Autodesk Fusion 360 part; units mm, degrees
(part 2 of 2)
sketch "スケッチ20" plane through (0, 0, 39.9) normal (0, 0, 1) x (1, 0, 0) in component "CASE_LID_print"
  line L0 (0.01, -5.9596) -> (0.01, -3.5388)
  line L1 (0.01, -3.5388) -> (1.0436, -3.5388)
  line L2 (1.0436, -3.5388) -> (1.0436, -3.8652)
  line L3 (1.0436, -3.8652) -> (0.3568, -3.8652)
  line L4 (0.3568, -3.8652) -> (0.3568, -4.5758)
  line L5 (0.3568, -4.5758) -> (0.9552, -4.5758)
  line L6 (0.9552, -4.5758) -> (0.9552, -4.9022)
  line L7 (0.9552, -4.9022) -> (0.3568, -4.9022)
  line L8 (0.3568, -4.9022) -> (0.3568, -5.6128)
  line L9 (0.3568, -5.6128) -> (1.0436, -5.6128)
  line L10 (1.0436, -5.6128) -> (1.0436, -5.9596)
  line L11 (1.0436, -5.9596) -> (0.01, -5.9596)
  line L12 (1.268, -5.9596) -> (1.268, -3.5388)
  line L13 (1.268, -3.5388) -> (1.6012, -3.5388)
  line L14 (1.6012, -3.5388) -> (2.0466, -4.8206)
  line L15 (2.0466, -4.8206) -> (2.0534, -4.8206)
  line L16 (2.0534, -4.8206) -> (2.4954, -3.5388)
  line L17 (2.4954, -3.5388) -> (2.832, -3.5388)
  line L18 (2.832, -3.5388) -> (2.832, -5.9596)
  line L19 (2.832, -5.9596) -> (2.4852, -5.9596)
  line L20 (2.4852, -5.9596) -> (2.4852, -4.4874)
  line L21 (2.4852, -4.4874) -> (2.4784, -4.4874)
  line L22 (2.4784, -4.4874) -> (2.135, -5.5278)
  line L23 (2.135, -5.5278) -> (1.9616, -5.5278)
  line L24 (1.9616, -5.5278) -> (1.6216, -4.4874)
  line L25 (1.6216, -4.4874) -> (1.6148, -4.4874)
  line L26 (1.6148, -4.4874) -> (1.6148, -5.9596)
  line L27 (1.6148, -5.9596) -> (1.268, -5.9596)
  line L28 (3.1584, -5.9596) -> (3.1584, -3.5388)
  line L29 (3.1584, -3.5388) -> (4.192, -3.5388)
  line L30 (4.192, -3.5388) -> (4.192, -3.8652)
  line L31 (4.192, -3.8652) -> (3.5052, -3.8652)
  line L32 (3.5052, -3.8652) -> (3.5052, -4.5758)
  line L33 (3.5052, -4.5758) -> (4.1036, -4.5758)
  line L34 (4.1036, -4.5758) -> (4.1036, -4.9022)
  line L35 (4.1036, -4.9022) -> (3.5052, -4.9022)
  line L36 (3.5052, -4.9022) -> (3.5052, -5.6128)
  line L37 (3.5052, -5.6128) -> (4.192, -5.6128)
  line L38 (4.192, -5.6128) -> (4.192, -5.9596)
  line L39 (4.192, -5.9596) -> (3.1584, -5.9596)
  line L40 (4.7632, -3.8652) -> (4.7632, -4.62)
  line L41 (4.7632, -4.62) -> (4.9604, -4.62)
  spline S0 degree 3 poles (4.9604, -4.62) (4.9881, -4.6195) (5.0381, -4.6187) (5.0855, -4.6031) (5.1066, -4.5962) knots 0 0 0 0 0.008266 0.014887 0.014887 0.014887 0.014887
  spline S1 degree 3 poles (5.1066, -4.5962) (5.1236, -4.5864) (5.1571, -4.5673) (5.1802, -4.5365) (5.1916, -4.5214) knots 0 0 0 0 0.005823 0.011428 0.011428 0.011428 0.011428
  spline S2 degree 3 poles (5.1916, -4.5214) (5.2, -4.5041) (5.218, -4.4674) (5.2252, -4.4271) (5.229, -4.4058) knots 0 0 0 0 0.005748 0.012202 0.012202 0.012202 0.012202
  spline S3 degree 3 poles (5.229, -4.4058) (5.232, -4.3803) (5.2383, -4.3261) (5.2389, -4.2715) (5.2392, -4.2426) knots 0 0 0 0 0.007688 0.016362 0.016362 0.016362 0.016362
  spline S4 degree 3 poles (5.2392, -4.2426) (5.2389, -4.2139) (5.2384, -4.1605) (5.232, -4.1074) (5.229, -4.0828) knots 0 0 0 0 0.008589 0.016023 0.016023 0.016023 0.016023
  spline S5 degree 3 poles (5.229, -4.0828) (5.225, -4.0603) (5.2174, -4.0175) (5.1976, -3.9788) (5.1882, -3.9604) knots 0 0 0 0 0.006804 0.012967 0.012967 0.012967 0.012967
  spline S6 degree 3 poles (5.1882, -3.9604) (5.1587, -3.9328) (5.0907, -3.8691) (4.9966, -3.8666) (4.9434, -3.8652) knots 0 0 0 0 0.011764 0.02708 0.02708 0.02708 0.02708
  line L42 (4.9434, -3.8652) -> (4.7632, -3.8652)
  line L43 (4.4164, -5.9596) -> (4.4164, -3.5388)
  line L44 (4.4164, -3.5388) -> (4.974, -3.5388)
  spline S7 degree 3 poles (4.974, -3.5388) (5.1523, -3.5749) (5.5316, -3.6516) (5.5671, -4.0424) (5.586, -4.2494) knots 0 0 0 0 0.049218 0.104666 0.104666 0.104666 0.104666
  spline S8 degree 3 poles (5.586, -4.2494) (5.584, -4.3161) (5.5803, -4.4411) (5.5378, -4.5585) (5.518, -4.6132) knots 0 0 0 0 0.019878 0.03722 0.03722 0.03722 0.03722
  spline S9 degree 3 poles (5.518, -4.6132) (5.4911, -4.6612) (5.435, -4.7615) (5.3376, -4.8227) (5.2868, -4.8546) knots 0 0 0 0 0.016243 0.033906 0.033906 0.033906 0.033906
  line L45 (5.2868, -4.8546) -> (5.6608, -5.9596)
  line L46 (5.6608, -5.9596) -> (5.2936, -5.9596)
  line L47 (5.2936, -5.9596) -> (4.9706, -4.926)
  line L48 (4.9706, -4.926) -> (4.7632, -4.926)
  line L49 (4.7632, -4.926) -> (4.7632, -5.9596)
  line L50 (4.7632, -5.9596) -> (4.4164, -5.9596)
  spline S10 degree 3 poles (5.8444, -4.11) (5.8461, -4.0636) (5.8494, -3.9747) (5.8805, -3.8914) (5.8954, -3.8516) knots 0 0 0 0 0.013829 0.02649 0.02649 0.02649 0.02649
  spline S11 degree 3 poles (5.8954, -3.8516) (5.9135, -3.816) (5.9489, -3.7465) (6.0043, -3.6915) (6.0314, -3.6646) knots 0 0 0 0 0.011882 0.023255 0.023255 0.023255 0.023255
  spline S12 degree 3 poles (6.0314, -3.6646) (6.0595, -3.6422) (6.1156, -3.5974) (6.1819, -3.5697) (6.215, -3.5558) knots 0 0 0 0 0.010711 0.021434 0.021434 0.021434 0.021434
  spline S13 degree 3 poles (6.215, -3.5558) (6.2499, -3.5449) (6.3185, -3.5234) (6.3904, -3.5201) (6.4258, -3.5184) knots 0 0 0 0 0.010907 0.021488 0.021488 0.021488 0.021488
  spline S14 degree 3 poles (6.4258, -3.5184) (6.4609, -3.52) (6.5317, -3.5232) (6.5992, -3.5449) (6.6332, -3.5558) knots 0 0 0 0 0.010497 0.021157 0.021157 0.021157 0.021157
  spline S15 degree 3 poles (6.6332, -3.5558) (6.6675, -3.5697) (6.7358, -3.5973) (6.7944, -3.6422) (6.8236, -3.6646) knots 0 0 0 0 0.01103 0.022019 0.022019 0.022019 0.022019
  spline S16 degree 3 poles (6.8236, -3.6646) (6.8497, -3.6916) (6.9035, -3.7471) (6.9383, -3.8161) (6.9562, -3.8516) knots 0 0 0 0 0.011203 0.023042 0.023042 0.023042 0.023042
  spline S17 degree 3 poles (6.9562, -3.8516) (6.9711, -3.8914) (7.0022, -3.9747) (7.0055, -4.0636) (7.0072, -4.11) knots 0 0 0 0 0.012662 0.02649 0.02649 0.02649 0.02649
  line L51 (7.0072, -4.11) -> (7.0072, -4.2324)
  line L52 (7.0072, -4.2324) -> (6.6604, -4.2324)
  line L53 (6.6604, -4.2324) -> (6.6604, -4.11)
  spline S18 degree 3 poles (6.6604, -4.11) (6.6587, -4.072) (6.6555, -4.0023) (6.6098, -3.9501) (6.589, -3.9264) knots 0 0 0 0 0.011025 0.020225 0.020225 0.020225 0.020225
  spline S19 degree 3 poles (6.589, -3.9264) (6.565, -3.9086) (6.5166, -3.8725) (6.4563, -3.8676) (6.4258, -3.8652) knots 0 0 0 0 0.008776 0.017747 0.017747 0.017747 0.017747
  spline S20 degree 3 poles (6.4258, -3.8652) (6.3951, -3.8677) (6.3339, -3.8727) (6.284, -3.9086) (6.2592, -3.9264) knots 0 0 0 0 0.009055 0.01805 0.01805 0.01805 0.01805
  spline S21 degree 3 poles (6.2592, -3.9264) (6.2394, -3.9502) (6.1956, -4.0031) (6.1927, -4.0721) (6.1912, -4.11) knots 0 0 0 0 0.009053 0.020065 0.020065 0.020065 0.020065
  line L54 (6.1912, -4.11) -> (6.1912, -5.3884)
  spline S22 degree 3 poles (6.1912, -5.3884) (6.1929, -5.4265) (6.1959, -5.4964) (6.2394, -5.5507) (6.2592, -5.5754) knots 0 0 0 0 0.011096 0.020361 0.020361 0.020361 0.020361
  spline S23 degree 3 poles (6.2592, -5.5754) (6.2841, -5.5923) (6.3345, -5.6263) (6.3952, -5.6309) (6.4258, -5.6332) knots 0 0 0 0 0.008867 0.017908 0.017908 0.017908 0.017908
  spline S24 degree 3 poles (6.4258, -5.6332) (6.4562, -5.631) (6.5159, -5.6266) (6.5649, -5.5923) (6.589, -5.5754) knots 0 0 0 0 0.008957 0.017603 0.017603 0.017603 0.017603
  spline S25 degree 3 poles (6.589, -5.5754) (6.6098, -5.5508) (6.6551, -5.4972) (6.6585, -5.4266) (6.6604, -5.3884) knots 0 0 0 0 0.009408 0.020517 0.020517 0.020517 0.020517
  line L55 (6.6604, -5.3884) -> (6.6604, -4.9328)
  line L56 (6.6604, -4.9328) -> (6.385, -4.9328)
  line L57 (6.385, -4.9328) -> (6.385, -4.6268)
  line L58 (6.385, -4.6268) -> (7.0072, -4.6268)
  line L59 (7.0072, -4.6268) -> (7.0072, -5.3884)
  spline S26 degree 3 poles (7.0072, -5.3884) (7.0057, -5.4363) (7.0028, -5.5264) (6.9711, -5.6107) (6.9562, -5.6502) knots 0 0 0 0 0.014252 0.026833 0.026833 0.026833 0.026833
  spline S27 degree 3 poles (6.9562, -5.6502) (6.9383, -5.6846) (6.9034, -5.7515) (6.8497, -5.8046) (6.8236, -5.8304) knots 0 0 0 0 0.011546 0.022495 0.022495 0.022495 0.022495
  spline S28 degree 3 poles (6.8236, -5.8304) (6.7945, -5.8538) (6.7364, -5.9003) (6.6675, -5.9285) (6.6332, -5.9426) knots 0 0 0 0 0.011136 0.022202 0.022202 0.022202 0.022202
  spline S29 degree 3 poles (6.6332, -5.9426) (6.5992, -5.9535) (6.5317, -5.9752) (6.4609, -5.9784) (6.4258, -5.98) knots 0 0 0 0 0.010661 0.021157 0.021157 0.021157 0.021157
  spline S30 degree 3 poles (6.4258, -5.98) (6.3904, -5.9783) (6.3185, -5.975) (6.2499, -5.9535) (6.215, -5.9426) knots 0 0 0 0 0.010581 0.021488 0.021488 0.021488 0.021488
  spline S31 degree 3 poles (6.215, -5.9426) (6.1818, -5.9285) (6.115, -5.9002) (6.0594, -5.8537) (6.0314, -5.8304) knots 0 0 0 0 0.010759 0.021622 0.021622 0.021622 0.021622
  spline S32 degree 3 poles (6.0314, -5.8304) (6.0043, -5.8047) (5.949, -5.7522) (5.9135, -5.6847) (5.8954, -5.6502) knots 0 0 0 0 0.011123 0.022712 0.022712 0.022712 0.022712
  spline S33 degree 3 poles (5.8954, -5.6502) (5.8805, -5.6107) (5.8488, -5.5264) (5.8459, -5.4363) (5.8444, -5.3884) knots 0 0 0 0 0.012581 0.026833 0.026833 0.026833 0.026833
  line L60 (5.8444, -5.3884) -> (5.8444, -4.11)
  line L61 (7.3132, -5.9596) -> (7.3132, -3.5388)
  line L62 (7.3132, -3.5388) -> (8.3468, -3.5388)
  line L63 (8.3468, -3.5388) -> (8.3468, -3.8652)
  line L64 (8.3468, -3.8652) -> (7.66, -3.8652)
  line L65 (7.66, -3.8652) -> (7.66, -4.5758)
  line L66 (7.66, -4.5758) -> (8.2584, -4.5758)
  line L67 (8.2584, -4.5758) -> (8.2584, -4.9022)
  line L68 (8.2584, -4.9022) -> (7.66, -4.9022)
  line L69 (7.66, -4.9022) -> (7.66, -5.6128)
  line L70 (7.66, -5.6128) -> (8.3468, -5.6128)
  line L71 (8.3468, -5.6128) -> (8.3468, -5.9596)
  line L72 (8.3468, -5.9596) -> (7.3132, -5.9596)
  line L73 (8.5576, -5.9596) -> (8.5576, -3.5388)
  line L74 (8.5576, -3.5388) -> (8.8908, -3.5388)
  line L75 (8.8908, -3.5388) -> (9.4144, -4.9974)
  line L76 (9.4144, -4.9974) -> (9.4212, -4.9974)
  line L77 (9.4212, -4.9974) -> (9.4212, -3.5388)
  line L78 (9.4212, -3.5388) -> (9.768, -3.5388)
  line L79 (9.768, -3.5388) -> (9.768, -5.9596)
  line L80 (9.768, -5.9596) -> (9.4416, -5.9596)
  line L81 (9.4416, -5.9596) -> (8.9112, -4.5044)
  line L82 (8.9112, -4.5044) -> (8.9044, -4.5044)
  line L83 (8.9044, -4.5044) -> (8.9044, -5.9596)
  line L84 (8.9044, -5.9596) -> (8.5576, -5.9596)
  line L85 (11.1824, -5.2694) -> (11.1824, -5.419)
  spline S34 degree 3 poles (11.1824, -5.419) (11.1806, -5.4559) (11.1769, -5.5296) (11.1511, -5.5987) (11.1382, -5.6332) knots 0 0 0 0 0.011021 0.021988 0.021988 0.021988 0.021988
  spline S35 degree 3 poles (11.1382, -5.6332) (11.1231, -5.6653) (11.0929, -5.7296) (11.0461, -5.7831) (11.0226, -5.81) knots 0 0 0 0 0.01057 0.021217 0.021217 0.021217 0.021217
  spline S36 degree 3 poles (11.0226, -5.81) (10.9964, -5.8349) (10.9434, -5.8851) (10.8785, -5.9188) (10.8458, -5.9358) knots 0 0 0 0 0.010787 0.021794 0.021794 0.021794 0.021794
  spline S37 degree 3 poles (10.8458, -5.9358) (10.8119, -5.9487) (10.7429, -5.9749) (10.6691, -5.9783) (10.6316, -5.98) knots 0 0 0 0 0.010806 0.021996 0.021996 0.021996 0.021996
  spline S38 degree 3 poles (10.6316, -5.98) (10.5983, -5.9788) (10.5306, -5.9763) (10.4646, -5.9607) (10.431, -5.9528) knots 0 0 0 0 0.009968 0.020287 0.020287 0.020287 0.020287
  spline S39 degree 3 poles (10.431, -5.9528) (10.3978, -5.942) (10.3314, -5.9204) (10.2754, -5.8786) (10.2474, -5.8576) knots 0 0 0 0 0.010387 0.020807 0.020807 0.020807 0.020807
  spline S40 degree 3 poles (10.2474, -5.8576) (10.2211, -5.8329) (10.1669, -5.7821) (10.1303, -5.7174) (10.1114, -5.6842) knots 0 0 0 0 0.01076 0.022149 0.022149 0.022149 0.022149
  spline S41 degree 3 poles (10.1114, -5.6842) (10.0966, -5.6435) (10.0641, -5.5547) (10.0617, -5.4601) (10.0604, -5.4088) knots 0 0 0 0 0.012905 0.028173 0.028173 0.028173 0.028173
  line L86 (10.0604, -5.4088) -> (10.0604, -4.076)
  spline S42 degree 3 poles (10.0604, -4.076) (10.062, -4.0374) (10.065, -3.9618) (10.0893, -3.8901) (10.1012, -3.855) knots 0 0 0 0 0.01152 0.022577 0.022577 0.022577 0.022577
  spline S43 degree 3 poles (10.1012, -3.855) (10.1161, -3.8223) (10.1456, -3.7574) (10.1932, -3.7044) (10.2168, -3.6782) knots 0 0 0 0 0.010721 0.021235 0.021235 0.021235 0.021235
  spline S44 degree 3 poles (10.2168, -3.6782) (10.243, -3.6546) (10.296, -3.607) (10.3609, -3.5775) (10.3936, -3.5626) knots 0 0 0 0 0.010514 0.021235 0.021235 0.021235 0.021235
  spline S45 degree 3 poles (10.3936, -3.5626) (10.4301, -3.5497) (10.5049, -3.5233) (10.5842, -3.5201) (10.6248, -3.5184) knots 0 0 0 0 0.011537 0.023657 0.023657 0.023657 0.023657
  spline S46 degree 3 poles (10.6248, -3.5184) (10.7018, -3.5243) (10.8515, -3.5357) (10.9667, -3.6316) (11.0226, -3.6782) knots 0 0 0 0 0.022542 0.043831 0.043831 0.043831 0.043831
  spline S47 degree 3 poles (11.0226, -3.6782) (11.0462, -3.7059) (11.0944, -3.7622) (11.1234, -3.8305) (11.1382, -3.8652) knots 0 0 0 0 0.010847 0.0221 0.0221 0.0221 0.0221
  spline S48 degree 3 poles (11.1382, -3.8652) (11.1511, -3.9017) (11.1775, -3.9765) (11.1807, -4.0558) (11.1824, -4.0964) knots 0 0 0 0 0.011536 0.023657 0.023657 0.023657 0.023657
  line L87 (11.1824, -4.0964) -> (11.1824, -4.2324)
  line L88 (11.1824, -4.2324) -> (10.8356, -4.2324)
  line L89 (10.8356, -4.2324) -> (10.8356, -4.1168)
  spline S49 degree 3 poles (10.8356, -4.1168) (10.8334, -4.0842) (10.8291, -4.0203) (10.7947, -3.9664) (10.7778, -3.94) knots 0 0 0 0 0.009629 0.018869 0.018869 0.018869 0.018869
  spline S50 degree 3 poles (10.7778, -3.94) (10.7566, -3.9182) (10.7138, -3.874) (10.6524, -3.8682) (10.6214, -3.8652) knots 0 0 0 0 0.008815 0.017851 0.017851 0.017851 0.017851
  spline S51 degree 3 poles (10.6214, -3.8652) (10.5829, -3.867) (10.5129, -3.8702) (10.4681, -3.9231) (10.448, -3.9468) knots 0 0 0 0 0.010986 0.019947 0.019947 0.019947 0.019947
  spline S52 degree 3 poles (10.448, -3.9468) (10.4361, -3.9762) (10.4102, -4.0404) (10.4082, -4.1098) (10.4072, -4.1474) knots 0 0 0 0 0.009435 0.020617 0.020617 0.020617 0.020617
  line L90 (10.4072, -4.1474) -> (10.4072, -5.385)
  spline S53 degree 3 poles (10.4072, -5.385) (10.4086, -5.4179) (10.4111, -5.48) (10.4385, -5.5356) (10.4514, -5.5618) knots 0 0 0 0 0.009753 0.018403 0.018403 0.018403 0.018403
  spline S54 degree 3 poles (10.4514, -5.5618) (10.4719, -5.5826) (10.5172, -5.6286) (10.5823, -5.6316) (10.618, -5.6332) knots 0 0 0 0 0.008456 0.018728 0.018728 0.018728 0.018728
  spline S55 degree 3 poles (10.618, -5.6332) (10.6297, -5.6327) (10.6538, -5.6317) (10.6773, -5.626) (10.6894, -5.623) knots 0 0 0 0 0.003494 0.007229 0.007229 0.007229 0.007229
  spline S56 degree 3 poles (10.6894, -5.623) (10.7027, -5.6179) (10.7295, -5.6076) (10.7526, -5.5907) (10.7642, -5.5822) knots 0 0 0 0 0.004264 0.008554 0.008554 0.008554 0.008554
  spline S57 degree 3 poles (10.7642, -5.5822) (10.7742, -5.5719) (10.7953, -5.5498) (10.8083, -5.5221) (10.8152, -5.5074) knots 0 0 0 0 0.004278 0.009108 0.009108 0.009108 0.009108
  spline S58 degree 3 poles (10.8152, -5.5074) (10.8211, -5.4897) (10.8341, -5.4511) (10.8351, -5.4104) (10.8356, -5.3884) knots 0 0 0 0 0.005569 0.012134 0.012134 0.012134 0.012134
  line L91 (10.8356, -5.3884) -> (10.8356, -5.2694)
  line L92 (10.8356, -5.2694) -> (11.1824, -5.2694)
  line L93 (11.7876, -5.9596) -> (11.7876, -4.9362)
  line L94 (11.7876, -4.9362) -> (11.3116, -3.5388)
  line L95 (11.3116, -3.5388) -> (11.6788, -3.5388)
  line L96 (11.6788, -3.5388) -> (11.9576, -4.501)
  line L97 (11.9576, -4.501) -> (11.9644, -4.501)
  line L98 (11.9644, -4.501) -> (12.2432, -3.5388)
  line L99 (12.2432, -3.5388) -> (12.6104, -3.5388)
  line L100 (12.6104, -3.5388) -> (12.1344, -4.9362)
  line L101 (12.1344, -4.9362) -> (12.1344, -5.9596)
  line L102 (12.1344, -5.9596) -> (11.7876, -5.9596)
extrude "押し出し39" add sketch "スケッチ20" along normal blind 0.8 separate body contours L0 L1 L2 L3 L4 L5 L6 L7 L8 L9 L10 L11 makes body 57 in component "CASE_LID_print"
extrude "押し出し40" add sketch "スケッチ20" along normal blind 0.8 separate body contours S10 S11 S12 S13 S14 S15 S16 S17 L51 L52 L53 S18 S19 S20 S21 L54 S22 S23 S24 S25 L55 L56 L57 L58 L59 S26 S27 S28 S29 S30 S31 S32 S33 L60 makes body 58 in component "CASE_LID_print"
extrude "押し出し41" add sketch "スケッチ20" along normal blind 0.8 separate body contours L61 L62 L63 L64 L65 L66 L67 L68 L69 L70 L71 L72 makes body 59 in component "CASE_LID_print"
extrude "押し出し42" add sketch "スケッチ20" along normal blind 0.8 separate body contours L40 L41 S0 S1 S2 S3 S4 S5 S6 L42 makes body 60 in component "CASE_LID_print"
extrude "押し出し43" add sketch "スケッチ20" along normal blind 0.8 separate body contours L43 L44 S7 S8 S9 L45 L46 L47 L48 L49 L50 makes body 61 in component "CASE_LID_print"
extrude "押し出し44" add sketch "スケッチ20" along normal blind 0.8 separate body contours L73 L74 L75 L76 L77 L78 L79 L80 L81 L82 L83 L84 makes body 62 in component "CASE_LID_print"
extrude "押し出し45" add sketch "スケッチ20" along normal blind 0.8 separate body contours L28 L29 L30 L31 L32 L33 L34 L35 L36 L37 L38 L39 makes body 63 in component "CASE_LID_print"
extrude "押し出し46" add sketch "スケッチ20" along normal blind 0.8 separate body contours L85 S34 S35 S36 S37 S38 S39 S40 S41 L86 S42 S43 S44 S45 S46 S47 S48 L87 L88 L89 S49 S50 S51 S52 L90 S53 S54 S55 S56 S57 S58 L91 L92 makes body 64 in component "CASE_LID_print"
extrude "押し出し47" add sketch "スケッチ20" along normal blind 0.8 separate body contours L12 L13 L14 L15 L16 L17 L18 L19 L20 L21 L22 L23 L24 L25 L26 L27 makes body 65 in component "CASE_LID_print"
extrude "押し出し48" add sketch "スケッチ20" along normal blind 0.8 separate body contours L93 L94 L95 L96 L97 L98 L99 L100 L101 L102 makes body 66 in component "CASE_LID_print"
move_body "移動2'" bodies 57 58 59 60 61 62 63 64 65 66 to x (1, 0, 0) y (0, 1, 0) z (0, 0, 1) at (-0.3102, 5.0492, 0) in component "CASE_LID_print"
combine "結合12'" operation add target body 19 tool bodies 57 58 59 60 61 62 63 64 65 66 in component "CASE_LID_print"
ref_plane "作業平面21" through (0, 0, 32.5) normal (0, 0, 1) x (1, 0, 0) in component "CASE_LID_print"
sketch "スケッチ21" plane through (0, 0, 32.5) normal (0, 0, 1) x (1, 0, 0) in component "CASE_LID_print"
  circle A0 centre (6, -18) radius 5.25
extrude "押し出し49" add sketch "スケッチ21" along normal blind 8.45 separate body makes body 67 in component "CASE_LID_print"
ref_plane "作業平面22" through (0, 0, 35) normal (0, 0, 1) x (1, 0, 0) in component "CASE_LID_print"
sketch "スケッチ22" plane through (0, 0, 35) normal (0, 0, 1) x (1, 0, 0) in component "CASE_LID_print"
  circle A0 centre (6, -18) radius 9.9
extrude "押し出し50" add sketch "スケッチ22" along normal blind 5.95 separate body makes body 68 in component "CASE_LID_print"
combine "結合13" operation cut target body 19 tool bodies 67 68 in component "CASE_LID_print"
ref_plane "作業平面1" through (0, 0, 37.6) normal (0, 0, 1) x (1, 0, 0) in component "EMERGENCY_BUTTON_PLUNGER_print"
sketch "スケッチ1 (3)" plane through (0, 0, 37.6) normal (0, 0, 1) x (1, 0, 0) in component "EMERGENCY_BUTTON_PLUNGER_print"
  circle A0 centre (6, -18) radius 9
extrude "押し出し1''" add sketch "スケッチ1 (3)" along normal blind 4 separate body makes body 69 in component "EMERGENCY_BUTTON_PLUNGER_print"
ref_plane "作業平面2" through (0, 0, 21.65) normal (0, 0, 1) x (1, 0, 0) in component "EMERGENCY_BUTTON_PLUNGER_print"
sketch "スケッチ2 (3)" plane through (0, 0, 21.65) normal (0, 0, 1) x (1, 0, 0) in component "EMERGENCY_BUTTON_PLUNGER_print"
  circle A0 centre (6, -18) radius 3.5
extrude "押し出し2''" add sketch "スケッチ2 (3)" along normal blind 15.95 separate body makes body 70 in component "EMERGENCY_BUTTON_PLUNGER_print"
combine "結合1''" operation add target body 69 tool bodies 70 in component "EMERGENCY_BUTTON_PLUNGER_print"
ref_plane "作業平面3" through (0, 0, 41.55) normal (0, 0, 1) x (1, 0, 0) in component "EMERGENCY_BUTTON_PLUNGER_print"
sketch "スケッチ3 (3)" plane through (0, 0, 41.55) normal (0, 0, 1) x (1, 0, 0) in component "EMERGENCY_BUTTON_PLUNGER_print"
  circle A0 centre (6, -18) radius 6.7
extrude "押し出し3''" add sketch "スケッチ3 (3)" along normal blind 0.55 separate body makes body 71 in component "EMERGENCY_BUTTON_PLUNGER_print"
ref_plane "作業平面4" through (0, 0, 41.45) normal (0, 0, 1) x (1, 0, 0) in component "EMERGENCY_BUTTON_PLUNGER_print"
sketch "スケッチ4 (3)" plane through (0, 0, 41.45) normal (0, 0, 1) x (1, 0, 0) in component "EMERGENCY_BUTTON_PLUNGER_print"
  circle A0 centre (6, -18) radius 5.2
extrude "押し出し4''" add sketch "スケッチ4 (3)" along normal blind 0.85 separate body makes body 72 in component "EMERGENCY_BUTTON_PLUNGER_print"
combine "結合2''" operation cut target body 71 tool bodies 72 in component "EMERGENCY_BUTTON_PLUNGER_print"
combine "結合3''" operation add target body 69 tool bodies 71 in component "EMERGENCY_BUTTON_PLUNGER_print"
ref_plane "作業平面5" through (0, 0, 41.55) normal (0, 0, 1) x (1, 0, 0) in component "EMERGENCY_BUTTON_PLUNGER_print"
sketch "スケッチ5 (3)" plane through (0, 0, 41.55) normal (0, 0, 1) x (1, 0, 0) in component "EMERGENCY_BUTTON_PLUNGER_print"
  line L0 (1.3541, -16.4787) -> (1.1543, -20.1691)
  line L1 (1.1543, -20.1691) -> (0.2098, -20.1691)
  line L2 (0.2098, -20.1691) -> (0.01, -16.4787)
  line L3 (0.01, -16.4787) -> (1.3541, -16.4787)
  line L4 (1.2542, -20.3991) -> (1.2542, -21.38)
  line L5 (1.2542, -21.38) -> (0.1099, -21.38)
  line L6 (0.1099, -21.38) -> (0.1099, -20.3991)
  line L7 (0.1099, -20.3991) -> (1.2542, -20.3991)
extrude "押し出し5''" add sketch "スケッチ5 (3)" along normal blind 0.6 separate body contours L0 L1 L2 L3 makes body 73 in component "EMERGENCY_BUTTON_PLUNGER_print"
extrude "押し出し6''" add sketch "スケッチ5 (3)" along normal blind 0.6 separate body contours L4 L5 L6 L7 makes body 74 in component "EMERGENCY_BUTTON_PLUNGER_print"
move_body "移動1''" bodies 73 74 to x (1, 0, 0) y (0, 1, 0) z (0, 0, 1) at (5.3179, 0.8294, 0) in component "EMERGENCY_BUTTON_PLUNGER_print"
combine "結合4''" operation add target body 69 tool bodies 73 74 in component "EMERGENCY_BUTTON_PLUNGER_print"
ref_plane "作業平面1" through (0, 0, 17.5) normal (0, 0, 1) x (1, 0, 0) in component "HARDWARE_REFERENCE_do_not_print"
sketch "スケッチ1 (4)" plane through (0, 0, 17.5) normal (0, 0, 1) x (1, 0, 0) in component "HARDWARE_REFERENCE_do_not_print"
  line L0 (-6, -28) -> (46, -28)
  line L1 (46, -28) -> (46, 32)
  line L2 (46, 32) -> (-6, 32)
  line L3 (-6, 32) -> (-6, -28)
extrude "押し出し1'''" add sketch "スケッチ1 (4)" along normal blind 15 separate body makes body 75 in component "HARDWARE_REFERENCE_do_not_print"
ref_plane "作業平面2" through (0, 0, 0) normal (0, 0, 1) x (1, 0, 0) in component "HARDWARE_REFERENCE_do_not_print"
sketch "スケッチ2 (4)" plane through (0, 0, 0) normal (0, 0, 1) x (1, 0, 0) in component "HARDWARE_REFERENCE_do_not_print"
  circle A0 centre (-22, -14) radius 25
extrude "押し出し2'''" add sketch "スケッチ2 (4)" along normal blind 12 separate body makes body 76 in component "HARDWARE_REFERENCE_do_not_print"
ref_plane "作業平面3" through (0, 0, 17.7) normal (0, 0, 1) x (1, 0, 0) in component "HARDWARE_REFERENCE_do_not_print"
sketch "スケッチ3 (4)" plane through (0, 0, 17.7) normal (0, 0, 1) x (1, 0, 0) in component "HARDWARE_REFERENCE_do_not_print"
  circle A0 centre (6, -18) radius 3.5
extrude "押し出し3'''" add sketch "スケッチ3 (4)" along normal blind 3.8 separate body makes body 77 in component "HARDWARE_REFERENCE_do_not_print"
ref_plane "作業平面4" through (0, 0, 23.5) normal (0, 0, 1) x (1, 0, 0) in component "HARDWARE_REFERENCE_do_not_print"
sketch "スケッチ4 (4)" plane through (0, 0, 23.5) normal (0, 0, 1) x (1, 0, 0) in component "HARDWARE_REFERENCE_do_not_print"
  line L0 (31, -31.1) -> (41, -31.1)
  line L1 (41, -31.1) -> (41, -26.1)
  line L2 (41, -26.1) -> (31, -26.1)
  line L3 (31, -26.1) -> (31, -31.1)
extrude "押し出し4'''" add sketch "スケッチ4 (4)" along normal blind 4 separate body makes body 78 in component "HARDWARE_REFERENCE_do_not_print"
component "CASE_BASE_print" placed x (1, 0, 0) y (0, 1, 0) z (0, 0, 1) at (0, 0, 0)
component "CASE_LID_print" placed x (1, 0, 0) y (0, 1, 0) z (0, 0, 1) at (0, 0, 0)
component "EMERGENCY_BUTTON_PLUNGER_print" placed x (1, 0, 0) y (0, 1, 0) z (0, 0, 1) at (0, 0, 0)
component "HARDWARE_REFERENCE_do_not_print" placed x (1, 0, 0) y (0, 1, 0) z (0, 0, 1) at (0, 0, 0)
named bodies: "base_shell", "cut_inner_cavity", "cut_bottom_connector_fit", "connector_retaining_ring", "cut_connector_ring_inner", "cut_microb_side_window", "cut_typec_front_window", "typec_rounded_deep_cable_dock", "cut_typec_rounded_dock_center", "typec_right_chamfer_root_fill", "standoff_1", "cut_standoff_hole_1", "standoff_2", "cut_standoff_hole_2", "standoff_3", "cut_standoff_hole_3", "standoff_4", "cut_standoff_hole_4", "lid_top", "lid_inside_lip", "cut_lid_lip_center", "cut_button_through_hole", "cut_button_top_recess", "button_guide_outer", "cut_button_guide_inner", "brand_center_armor_plate", "left_upper_shoulder_plate", "right_upper_shoulder_plate", "left_lower_fang_plate", "right_lower_fang_plate", "emergency_octagonal_deck", "emergency_label_close_plate", "raised_brand_text_1", "raised_brand_text_2", "raised_brand_text_3", "raised_brand_text_4", "raised_brand_text_5", "raised_brand_text_6", "raised_brand_text_7", "raised_brand_text_8", "raised_brand_text_9", "raised_brand_text_10", "raised_brand_text_11", "raised_brand_text_12", "raised_brand_text_13", "raised_brand_text_14", "raised_brand_text_15", "raised_brand_text_16", "raised_brand_text_17", "raised_brand_text_18", "raised_brand_text_19", "raised_brand_text_20", "cut_five_mm_protective_edge_groove_outer", "cut_five_mm_protective_edge_groove_inner", "emergency_button_guard_ring_outer", "cut_emergency_button_guard_ring_inner", "raised_emergency_label_1", "raised_emergency_label_2", "raised_emergency_label_3", "raised_emergency_label_4", "raised_emergency_label_5", "raised_emergency_label_6", "raised_emergency_label_7", "raised_emergency_label_8", "raised_emergency_label_9", "raised_emergency_label_10", "cut_final_button_through_hole", "cut_final_button_top_recess", "button_cap_protruding_emergency", "button_stem_to_tact_switch", "button_tactile_top_ring_outer", "cut_button_tactile_top_ring_inner", "raised_button_bang_1", "raised_button_bang_2", "board_envelope_52x60x15", "connector_puck_50x12", "emergency_tact_switch_7mm", "typec_reference_10mm_high_mount"
